Autodesk Fusion 360 part; units mm, degrees
(part 2 of 2)
sketch "Skizze22" plane through (0, 0, 0) normal (0, 1, 0) x (1, 0, 0)
  circle A0 centre (300.5747, -360.375) radius 1.05
  circle A1 centre (290.8247, -423.625) radius 1.05
  circle A2 centre (342.5747, -360.375) radius 1.05
  circle A3 centre (300.5747, -410.375) radius 1.05
  circle A4 centre (352.3247, -423.625) radius 1.05
  circle A5 centre (290.8247, -347.125) radius 1.05
  circle A6 centre (342.5747, -410.375) radius 1.05
  circle A7 centre (352.3247, -347.125) radius 1.05
  line L0 (372.375, -423.1301) -> (372.375, -432.6968)
  line L1 (372.375, -443.625) -> (354.375, -443.625)
  line L2 (270.8247, -443.625) -> (270.8247, -437.3156)
  line L3 (270.8247, -437.3156) -> (274.8247, -439.625)
  line L4 (274.8247, -439.625) -> (278.8247, -437.3156)
  line L5 (278.8247, -437.3156) -> (278.8247, -432.6968)
  line L6 (278.8247, -432.6968) -> (274.8247, -430.3874)
  line L7 (274.8247, -430.3874) -> (270.8247, -432.6968)
  line L8 (270.8247, -432.6968) -> (270.8247, -423.1299)
  line L9 (270.8247, -333.4429) -> (270.8247, -327.125)
  line L10 (270.8247, -327.125) -> (288.875, -327.125)
  line L11 (372.375, -327.125) -> (372.375, -333.4372)
  line L12 (372.375, -338.0617) -> (372.375, -347.6245)
  line L13 (372.375, -347.6245) -> (365.5189, -347.6245)
  line L14 (365.5189, -347.6245) -> (352.7821, -385.3833)
  line L15 (352.7821, -385.3833) -> (365.5137, -423.1301)
  line L16 (365.5137, -423.1301) -> (372.375, -423.1301)
  circle A8 centre (352.3247, -347.125) radius 1.05
  circle A9 centre (342.5747, -410.375) radius 1.05
  circle A10 centre (290.8247, -347.125) radius 1.05
  circle A11 centre (352.3247, -423.625) radius 1.05
  circle A12 centre (300.5747, -410.375) radius 1.05
  circle A13 centre (342.5747, -360.375) radius 1.05
  circle A14 centre (290.8247, -423.625) radius 1.05
  circle A15 centre (300.5747, -360.375) radius 1.05
  line L17 (354.375, -443.625) -> (372.375, -443.625)
  line L18 (270.8247, -437.3156) -> (270.8247, -443.625)
  line L19 (270.8247, -437.3156) -> (274.8247, -439.625)
  line L20 (274.8247, -439.625) -> (278.8247, -437.3156)
  line L21 (278.8247, -437.3156) -> (278.8247, -432.6968)
  line L22 (278.8247, -432.6968) -> (274.8247, -430.3874)
  line L23 (274.8247, -430.3874) -> (270.8247, -432.6968)
  line L24 (270.8247, -423.1299) -> (270.8247, -432.6968)
  line L25 (270.8247, -327.125) -> (270.8247, -333.4429)
  line L26 (288.875, -327.125) -> (270.8247, -327.125)
  line L27 (372.375, -333.4372) -> (372.375, -327.125)
  line L28 (372.375, -347.6245) -> (372.375, -338.0617)
  line L29 (365.5189, -347.6245) -> (372.375, -347.6245)
  line L30 (352.7821, -385.3833) -> (365.5189, -347.6245)
  line L31 (365.5137, -423.1301) -> (352.7821, -385.3833)
  line L32 (372.375, -423.1301) -> (365.5137, -423.1301)
  line L33 (372.375, -432.6968) -> (372.375, -423.1301)
  line L34 (372.375, -333.4372) -> (376.3602, -331.125)
  line L35 (376.3602, -331.125) -> (380.3651, -333.4259)
  line L36 (380.3651, -333.4259) -> (380.375, -338.0447)
  line L37 (380.375, -338.0447) -> (376.3799, -340.3626)
  line L38 (376.3799, -340.3626) -> (372.375, -338.0617)
  arc A16 (176.5, -116.5) -> (180.5, -112.5) centre (180.5, -116.5) ccw
  line L39 (176.5, -116.5) -> (71.5, -116.5)
  arc A17 (67.5, -112.5) -> (71.5, -116.5) centre (67.5, -116.5) ccw
  line L40 (67.5, -112.5) -> (67.5, -95)
  arc A18 (67.5, -87) -> (67.5, -95) centre (67.5, -91) ccw
  line L41 (67.5, -87) -> (67.5, -69)
  arc A19 (71.5, -65) -> (67.5, -69) centre (67.5, -65) ccw
  line L42 (71.5, -65) -> (176.5, -65)
  arc A20 (180.5, -69) -> (176.5, -65) centre (180.5, -65) ccw
  line L43 (180.5, -69) -> (180.5, -87)
  arc A21 (180.5, -95) -> (180.5, -87) centre (180.5, -91) ccw
  line L44 (180.5, -95) -> (180.5, -112.5)
  line L45 (137.5, 7.5) -> (104.5, 7.5)
  line L46 (104.5, 7.5) -> (104.5, 23.5)
  line L47 (104.5, 23.5) -> (102, 23.5)
  line L48 (102, 23.5) -> (102, 34.5)
  line L49 (102, 34.5) -> (140, 34.5)
  line L50 (140, 34.5) -> (140, 23.5)
  line L51 (140, 23.5) -> (137.5, 23.5)
  line L52 (137.5, 23.5) -> (137.5, 7.5)
  line L53 (455, -207) -> (552.928, -207)
  line L54 (552.928, -207) -> (552.928, -27)
  line L55 (552.928, -27) -> (455, -27)
  line L56 (455, -27) -> (455, -207)
  line L57 (583, -14) -> (583, -27)
  line L58 (583, -27) -> (572.928, -27)
  line L59 (572.928, -27) -> (572.928, -207)
  line L60 (572.928, -207) -> (583, -207)
  line L61 (583, -207) -> (583, -225)
  line L62 (583, -225) -> (315, -225)
  line L63 (315, -225) -> (315, -14)
  line L64 (315, -14) -> (583, -14)
  line L65 (59, -3.5) -> (35, -3.5)
  line L66 (35, -3.5) -> (35, 34.5)
  line L67 (35, 34.5) -> (59, 34.5)
  line L68 (59, 34.5) -> (59, -3.5)
  line L69 (82, 4.5) -> (82, 34.5)
  line L70 (82, 34.5) -> (100, 34.5)
  line L71 (100, 34.5) -> (100, 4.5)
  line L72 (100, 4.5) -> (82, 4.5)
  circle A22 centre (386.2786, 261.3333) radius 3
  circle A23 centre (386.2786, 178.3693) radius 2
  line L73 (382.7786, 285.8333) -> (389.7786, 285.8333)
  line L74 (389.7786, 285.8333) -> (389.7786, 271.3333)
  line L75 (389.7786, 271.3333) -> (382.7786, 271.3333)
  line L76 (382.7786, 271.3333) -> (382.7786, 285.8333)
  line L77 (-65.5, -219) -> (-65.5, -239)
  line L78 (-65.5, -239) -> (-66.5, -239)
  line L79 (-66.5, -239) -> (-66.5, -219)
  line L80 (-66.5, -219) -> (-65.5, -219)
  circle A24 centre (115, 170.025) radius 2
  circle A25 centre (220, 275.025) radius 2
  circle A26 centre (115, 275.025) radius 2
  circle A27 centre (167.5, 222.525) radius 57.5
  circle A28 centre (220, 170.025) radius 2
  line L81 (92.5, 328.025) -> (242.5, 328.025)
  line L82 (242.5, 328.025) -> (242.5, 117.025)
  line L83 (242.5, 117.025) -> (92.5, 117.025)
  line L84 (92.5, 117.025) -> (92.5, 328.025)
  circle A29 centre (22, 160.025) radius 2
  circle A30 centre (-102, 160.025) radius 2
  circle A31 centre (-102, 284.025) radius 2
  circle A32 centre (22, 284.025) radius 2
  circle A33 centre (-40, 222.025) radius 67.5
  line L85 (-115, 327.525) -> (35, 327.525)
  line L86 (35, 327.525) -> (35, 116.525)
  line L87 (35, 116.525) -> (-115, 116.525)
  line L88 (-115, 116.525) -> (-115, 327.525)
  line L89 (190.5, -319) -> (190.5, -339)
  line L90 (190.5, -339) -> (189.5, -339)
  line L91 (189.5, -339) -> (189.5, -319)
  line L92 (189.5, -319) -> (190.5, -319)
  line L93 (198, -317) -> (182, -317)
  line L94 (182, -317) -> (182, -339.5)
  line L95 (182, -339.5) -> (-58, -339.5)
  line L96 (-58, -339.5) -> (-58, -219.5)
  line L97 (-58, -219.5) -> (182, -219.5)
  line L98 (182, -219.5) -> (182, -242)
  line L99 (182, -242) -> (198, -242)
  arc A34 (203, -247) -> (198, -242) centre (198, -247) ccw
  line L100 (203, -247) -> (203, -312)
  arc A35 (198, -317) -> (203, -312) centre (198, -312) ccw
  line L101 (382.7786, 235.3333) -> (389.7786, 235.3333)
  line L102 (389.7786, 235.3333) -> (389.7786, 220.8333)
  line L103 (389.7786, 220.8333) -> (382.7786, 220.8333)
  line L104 (382.7786, 220.8333) -> (382.7786, 235.3333)
  circle A36 centre (386.283, 172.3693) radius 3.5
  circle A37 centre (386.2786, 245.3333) radius 3
  circle A38 centre (386.2786, 162.3693) radius 4.5
  line L105 (78.5, 4.5) -> (60.5, 4.5)
  line L106 (60.5, 4.5) -> (60.5, 34.5)
  line L107 (60.5, 34.5) -> (78.5, 34.5)
  line L108 (78.5, 34.5) -> (78.5, 4.5)
  line L109 (28.5, 32) -> (28.5, -74)
  line L110 (28.5, -74) -> (35.5, -74)
  line L111 (35.5, -74) -> (35.5, -77)
  line L112 (35.5, -77) -> (-15.5, -77)
  line L113 (-15.5, -77) -> (-15.5, -74)
  line L114 (-15.5, -74) -> (-8.5, -74)
  line L115 (-8.5, -74) -> (-8.5, 32)
  line L116 (-8.5, 32) -> (28.5, 32)
  circle A39 centre (300.5747, -410.375) radius 1.05
  circle A40 centre (342.5747, -360.375) radius 1.05
  circle A41 centre (352.3247, -347.125) radius 1.05
  circle A42 centre (342.5747, -410.375) radius 1.05
  circle A43 centre (300.5747, -360.375) radius 1.05
  circle A44 centre (290.8247, -423.625) radius 1.05
  circle A45 centre (352.3247, -423.625) radius 1.05
  circle A46 centre (290.8247, -347.125) radius 1.05
  line L117 (270.8247, -443.625) -> (270.8247, -437.3156)
  line L118 (270.8247, -437.3156) -> (274.8247, -439.625)
  line L119 (274.8247, -439.625) -> (278.8247, -437.3156)
  line L120 (278.8247, -437.3156) -> (278.8247, -432.6968)
  line L121 (278.8247, -432.6968) -> (274.8247, -430.3874)
  line L122 (274.8247, -430.3874) -> (270.8247, -432.6968)
  line L123 (270.8247, -432.6968) -> (270.8247, -423.1299)
  line L124 (270.8247, -333.4429) -> (270.8247, -327.125)
  line L125 (270.8247, -327.125) -> (288.875, -327.125)
  line L126 (372.375, -327.125) -> (372.375, -333.4372)
  line L127 (372.375, -333.4372) -> (376.3602, -331.125)
  line L128 (376.3602, -331.125) -> (380.3651, -333.4259)
  line L129 (380.3651, -333.4259) -> (380.375, -338.0447)
  line L130 (380.375, -338.0447) -> (376.3799, -340.3626)
  line L131 (376.3799, -340.3626) -> (372.375, -338.0617)
  line L132 (372.375, -338.0617) -> (372.375, -347.6245)
  line L133 (372.375, -347.6245) -> (365.5189, -347.6245)
  line L134 (365.5189, -347.6245) -> (352.7821, -385.3833)
  line L135 (352.7821, -385.3833) -> (365.5137, -423.1301)
  line L136 (365.5137, -423.1301) -> (372.375, -423.1301)
  line L137 (372.375, -423.1301) -> (372.375, -432.6968)
  line L138 (372.375, -443.625) -> (354.375, -443.625)
  line L139 (-66.5, -319) -> (-65.5, -319)
  line L140 (-65.5, -319) -> (-65.5, -339)
  line L141 (-65.5, -339) -> (-66.5, -339)
  line L142 (-66.5, -339) -> (-66.5, -319)
  line L143 (189.5, -239) -> (189.5, -219)
  line L144 (189.5, -219) -> (190.5, -219)
  line L145 (190.5, -219) -> (190.5, -239)
  line L146 (190.5, -239) -> (189.5, -239)
  arc A47 (176.5, -116.5) -> (180.5, -112.5) centre (180.5, -116.5) ccw
  line L147 (176.5, -116.5) -> (71.5, -116.5)
  arc A48 (67.5, -112.5) -> (71.5, -116.5) centre (67.5, -116.5) ccw
  line L148 (67.5, -112.5) -> (67.5, -95)
  arc A49 (67.5, -87) -> (67.5, -95) centre (67.5, -91) ccw
  line L149 (67.5, -87) -> (67.5, -69)
  arc A50 (71.5, -65) -> (67.5, -69) centre (67.5, -65) ccw
  line L150 (71.5, -65) -> (176.5, -65)
  arc A51 (180.5, -69) -> (176.5, -65) centre (180.5, -65) ccw
  line L151 (180.5, -69) -> (180.5, -87)
  arc A52 (180.5, -95) -> (180.5, -87) centre (180.5, -91) ccw
  line L152 (180.5, -95) -> (180.5, -112.5)
  line L153 (137.5, 7.5) -> (104.5, 7.5)
  line L154 (104.5, 7.5) -> (104.5, 23.5)
  line L155 (104.5, 23.5) -> (102, 23.5)
  line L156 (102, 23.5) -> (102, 34.5)
  line L157 (102, 34.5) -> (140, 34.5)
  line L158 (140, 34.5) -> (140, 23.5)
  line L159 (140, 23.5) -> (137.5, 23.5)
  line L160 (137.5, 23.5) -> (137.5, 7.5)
  line L161 (455, -207) -> (552.928, -207)
  line L162 (552.928, -207) -> (552.928, -27)
  line L163 (552.928, -27) -> (455, -27)
  line L164 (455, -27) -> (455, -207)
  line L165 (583, -14) -> (583, -27)
  line L166 (583, -27) -> (572.928, -27)
  line L167 (572.928, -27) -> (572.928, -207)
  line L168 (572.928, -207) -> (583, -207)
  line L169 (583, -207) -> (583, -225)
  line L170 (583, -225) -> (315, -225)
  line L171 (315, -225) -> (315, -14)
  line L172 (315, -14) -> (583, -14)
  line L173 (59, -3.5) -> (35, -3.5)
  line L174 (35, -3.5) -> (35, 34.5)
  line L175 (35, 34.5) -> (59, 34.5)
  line L176 (59, 34.5) -> (59, -3.5)
  line L177 (82, 4.5) -> (82, 34.5)
  line L178 (82, 34.5) -> (100, 34.5)
  line L179 (100, 34.5) -> (100, 4.5)
  line L180 (100, 4.5) -> (82, 4.5)
  circle A53 centre (386.2786, 261.3333) radius 3
  circle A54 centre (386.2786, 178.3693) radius 2
  line L181 (382.7786, 285.8333) -> (389.7786, 285.8333)
  line L182 (389.7786, 285.8333) -> (389.7786, 271.3333)
  line L183 (389.7786, 271.3333) -> (382.7786, 271.3333)
  line L184 (382.7786, 271.3333) -> (382.7786, 285.8333)
  line L185 (-65.5, -219) -> (-65.5, -239)
  line L186 (-65.5, -239) -> (-66.5, -239)
  line L187 (-66.5, -239) -> (-66.5, -219)
  line L188 (-66.5, -219) -> (-65.5, -219)
  circle A55 centre (115, 170.025) radius 2
  circle A56 centre (220, 275.025) radius 2
  circle A57 centre (115, 275.025) radius 2
  circle A58 centre (167.5, 222.525) radius 57.5
  circle A59 centre (220, 170.025) radius 2
  line L189 (92.5, 328.025) -> (242.5, 328.025)
  line L190 (242.5, 328.025) -> (242.5, 117.025)
  line L191 (242.5, 117.025) -> (92.5, 117.025)
  line L192 (92.5, 117.025) -> (92.5, 328.025)
  circle A60 centre (22, 160.025) radius 2
  circle A61 centre (-102, 160.025) radius 2
  circle A62 centre (-102, 284.025) radius 2
  circle A63 centre (22, 284.025) radius 2
  circle A64 centre (-40, 222.025) radius 67.5
  line L193 (-115, 327.525) -> (35, 327.525)
  line L194 (35, 327.525) -> (35, 116.525)
  line L195 (35, 116.525) -> (-115, 116.525)
  line L196 (-115, 116.525) -> (-115, 327.525)
  line L197 (190.5, -319) -> (190.5, -339)
  line L198 (190.5, -339) -> (189.5, -339)
  line L199 (189.5, -339) -> (189.5, -319)
  line L200 (189.5, -319) -> (190.5, -319)
  line L201 (198, -317) -> (182, -317)
  line L202 (182, -317) -> (182, -339.5)
  line L203 (182, -339.5) -> (-58, -339.5)
  line L204 (-58, -339.5) -> (-58, -219.5)
  line L205 (-58, -219.5) -> (182, -219.5)
  line L206 (182, -219.5) -> (182, -242)
  line L207 (182, -242) -> (198, -242)
  arc A65 (203, -247) -> (198, -242) centre (198, -247) ccw
  line L208 (203, -247) -> (203, -312)
  arc A66 (198, -317) -> (203, -312) centre (198, -312) ccw
  line L209 (382.7786, 235.3333) -> (389.7786, 235.3333)
  line L210 (389.7786, 235.3333) -> (389.7786, 220.8333)
  line L211 (389.7786, 220.8333) -> (382.7786, 220.8333)
  line L212 (382.7786, 220.8333) -> (382.7786, 235.3333)
  circle A67 centre (386.283, 172.3693) radius 3.5
  circle A68 centre (386.2786, 245.3333) radius 3
  circle A69 centre (386.2786, 162.3693) radius 4.5
  line L213 (78.5, 4.5) -> (60.5, 4.5)
  line L214 (60.5, 4.5) -> (60.5, 34.5)
  line L215 (60.5, 34.5) -> (78.5, 34.5)
  line L216 (78.5, 34.5) -> (78.5, 4.5)
  line L217 (28.5, 32) -> (28.5, -74)
  line L218 (28.5, -74) -> (35.5, -74)
  line L219 (35.5, -74) -> (35.5, -77)
  line L220 (35.5, -77) -> (-15.5, -77)
  line L221 (-15.5, -77) -> (-15.5, -74)
  line L222 (-15.5, -74) -> (-8.5, -74)
  line L223 (-8.5, -74) -> (-8.5, 32)
  line L224 (-8.5, 32) -> (28.5, 32)
  circle A70 centre (300.5747, -410.375) radius 1.05
  circle A71 centre (342.5747, -360.375) radius 1.05
  circle A72 centre (352.3247, -347.125) radius 1.05
  circle A73 centre (342.5747, -410.375) radius 1.05
  circle A74 centre (300.5747, -360.375) radius 1.05
  circle A75 centre (290.8247, -423.625) radius 1.05
  circle A76 centre (352.3247, -423.625) radius 1.05
  circle A77 centre (290.8247, -347.125) radius 1.05
  line L225 (270.8247, -443.625) -> (270.8247, -437.3156)
  line L226 (270.8247, -437.3156) -> (274.8247, -439.625)
  line L227 (274.8247, -439.625) -> (278.8247, -437.3156)
  line L228 (278.8247, -437.3156) -> (278.8247, -432.6968)
  line L229 (278.8247, -432.6968) -> (274.8247, -430.3874)
  line L230 (274.8247, -430.3874) -> (270.8247, -432.6968)
  line L231 (270.8247, -432.6968) -> (270.8247, -423.1299)
  line L232 (270.8247, -333.4429) -> (270.8247, -327.125)
  line L233 (270.8247, -327.125) -> (288.875, -327.125)
  line L234 (372.375, -327.125) -> (372.375, -333.4372)
  line L235 (372.375, -333.4372) -> (376.3602, -331.125)
  line L236 (376.3602, -331.125) -> (380.3651, -333.4259)
  line L237 (380.3651, -333.4259) -> (380.375, -338.0447)
  line L238 (380.375, -338.0447) -> (376.3799, -340.3626)
  line L239 (376.3799, -340.3626) -> (372.375, -338.0617)
  line L240 (372.375, -338.0617) -> (372.375, -347.6245)
  line L241 (372.375, -347.6245) -> (365.5189, -347.6245)
  line L242 (365.5189, -347.6245) -> (352.7821, -385.3833)
  line L243 (352.7821, -385.3833) -> (365.5137, -423.1301)
  line L244 (365.5137, -423.1301) -> (372.375, -423.1301)
  line L245 (372.375, -423.1301) -> (372.375, -432.6968)
  line L246 (372.375, -443.625) -> (354.375, -443.625)
  line L247 (-66.5, -319) -> (-65.5, -319)
  line L248 (-65.5, -319) -> (-65.5, -339)
  line L249 (-65.5, -339) -> (-66.5, -339)
  line L250 (-66.5, -339) -> (-66.5, -319)
  line L251 (189.5, -239) -> (189.5, -219)
  line L252 (189.5, -219) -> (190.5, -219)
  line L253 (190.5, -219) -> (190.5, -239)
  line L254 (190.5, -239) -> (189.5, -239)
  line L255 (376.3602, -331.125) -> (372.375, -333.4372)
  line L256 (380.3651, -333.4259) -> (376.3602, -331.125)
  line L257 (380.375, -338.0447) -> (380.3651, -333.4259)
  line L258 (376.3799, -340.3626) -> (380.375, -338.0447)
  line L259 (372.375, -338.0617) -> (376.3799, -340.3626)
  line L260 (274.8394, -340.3626) -> (278.8345, -338.0447)
  line L261 (278.8345, -338.0447) -> (278.8247, -333.4259)
  line L262 (278.8247, -333.4259) -> (274.8198, -331.125)
  line L263 (274.8198, -331.125) -> (270.8247, -333.4429)
  line L264 (270.8247, -333.4429) -> (270.8345, -338.0617)
  line L265 (270.8345, -338.0617) -> (274.8394, -340.3626)
  line L266 (372.375, -432.6968) -> (376.375, -430.3874)
  line L267 (376.375, -430.3874) -> (380.375, -432.6968)
  line L268 (380.375, -432.6968) -> (380.375, -437.3156)
  line L269 (380.375, -437.3156) -> (376.375, -439.625)
  line L270 (376.375, -439.625) -> (372.375, -437.3156)
  line L271 (372.375, -437.3156) -> (372.375, -443.625)
  line L272 (274.8394, -340.3626) -> (278.8345, -338.0447)
  line L273 (278.8345, -338.0447) -> (278.8247, -333.4259)
  line L274 (278.8247, -333.4259) -> (274.8198, -331.125)
  line L275 (274.8198, -331.125) -> (270.8247, -333.4429)
  line L276 (270.8247, -333.4429) -> (270.8345, -338.0617)
  line L277 (270.8345, -338.0617) -> (274.8394, -340.3626)
  line L278 (372.375, -432.6968) -> (376.375, -430.3874)
  line L279 (376.375, -430.3874) -> (380.375, -432.6968)
  line L280 (380.375, -432.6968) -> (380.375, -437.3156)
  line L281 (380.375, -437.3156) -> (376.375, -439.625)
  line L282 (376.375, -439.625) -> (372.375, -437.3156)
  line L283 (372.375, -437.3156) -> (372.375, -443.625)
  line L284 (274.8394, -340.3626) -> (278.8345, -338.0447)
  line L285 (278.8345, -338.0447) -> (278.8247, -333.4259)
  line L286 (278.8247, -333.4259) -> (274.8198, -331.125)
  line L287 (274.8198, -331.125) -> (270.8247, -333.4429)
  line L288 (270.8247, -333.4429) -> (270.8345, -338.0617)
  line L289 (270.8345, -338.0617) -> (274.8394, -340.3626)
  line L290 (372.375, -432.6968) -> (376.375, -430.3874)
  line L291 (376.375, -430.3874) -> (380.375, -432.6968)
  line L292 (380.375, -432.6968) -> (380.375, -437.3156)
  line L293 (380.375, -437.3156) -> (376.375, -439.625)
  line L294 (376.375, -439.625) -> (372.375, -437.3156)
  line L295 (372.375, -437.3156) -> (372.375, -443.625)
  line L296 (278.8345, -338.0447) -> (278.8247, -333.4259)
  line L297 (278.8247, -333.4259) -> (274.8198, -331.125)
  line L298 (274.8198, -331.125) -> (270.8247, -333.4429)
  line L299 (270.8247, -333.4429) -> (270.8345, -338.0617)
  line L300 (270.8345, -338.0617) -> (274.8394, -340.3626)
  line L301 (274.8394, -340.3626) -> (278.8345, -338.0447)
  line L302 (376.375, -430.3874) -> (372.375, -432.6968)
  line L303 (380.375, -432.6968) -> (376.375, -430.3874)
  line L304 (380.375, -437.3156) -> (380.375, -432.6968)
  line L305 (376.375, -439.625) -> (380.375, -437.3156)
  line L306 (372.375, -437.3156) -> (376.375, -439.625)
  line L307 (372.375, -443.625) -> (372.375, -437.3156)
  line L308 (270.8247, -423.1299) -> (277.6357, -423.1301)
  line L309 (277.6357, -423.1301) -> (290.3673, -385.3833)
  line L310 (290.3673, -385.3833) -> (277.6305, -347.6245)
  line L311 (277.6305, -347.6245) -> (270.8247, -347.6245)
  line L312 (270.8247, -347.6245) -> (270.8247, -333.4429)
  line L313 (288.875, -327.125) -> (288.875, -336.084)
  line L314 (288.875, -336.084) -> (321.625, -343.6621)
  line L315 (321.625, -343.6621) -> (354.375, -336.084)
  line L316 (354.375, -336.084) -> (354.375, -327.125)
  line L317 (354.375, -327.125) -> (372.375, -327.125)
  line L318 (354.375, -443.625) -> (354.375, -434.666)
  line L319 (354.375, -434.666) -> (321.625, -427.088)
  line L320 (321.625, -427.088) -> (288.875, -434.666)
  line L321 (288.875, -434.666) -> (288.875, -443.625)
  line L322 (288.875, -443.625) -> (270.8247, -443.625)
  line L323 (270.8247, -423.1299) -> (277.6357, -423.1301)
  line L324 (277.6357, -423.1301) -> (290.3673, -385.3833)
  line L325 (290.3673, -385.3833) -> (277.6305, -347.6245)
  line L326 (277.6305, -347.6245) -> (270.8247, -347.6245)
  line L327 (270.8247, -347.6245) -> (270.8247, -333.4429)
  line L328 (288.875, -327.125) -> (288.875, -336.084)
  line L329 (288.875, -336.084) -> (321.625, -343.6621)
  line L330 (321.625, -343.6621) -> (354.375, -336.084)
  line L331 (354.375, -336.084) -> (354.375, -327.125)
  line L332 (354.375, -327.125) -> (372.375, -327.125)
  line L333 (354.375, -443.625) -> (354.375, -434.666)
  line L334 (354.375, -434.666) -> (321.625, -427.088)
  line L335 (321.625, -427.088) -> (288.875, -434.666)
  line L336 (288.875, -434.666) -> (288.875, -443.625)
  line L337 (288.875, -443.625) -> (270.8247, -443.625)
  line L338 (270.8247, -423.1299) -> (277.6357, -423.1301)
  line L339 (277.6357, -423.1301) -> (290.3673, -385.3833)
  line L340 (290.3673, -385.3833) -> (277.6305, -347.6245)
  line L341 (277.6305, -347.6245) -> (270.8247, -347.6245)
  line L342 (270.8247, -347.6245) -> (270.8247, -333.4429)
  line L343 (288.875, -327.125) -> (288.875, -336.084)
  line L344 (288.875, -336.084) -> (321.625, -343.6621)
  line L345 (321.625, -343.6621) -> (354.375, -336.084)
  line L346 (354.375, -336.084) -> (354.375, -327.125)
  line L347 (354.375, -327.125) -> (372.375, -327.125)
  line L348 (354.375, -443.625) -> (354.375, -434.666)
  line L349 (354.375, -434.666) -> (321.625, -427.088)
  line L350 (321.625, -427.088) -> (288.875, -434.666)
  line L351 (288.875, -434.666) -> (288.875, -443.625)
  line L352 (288.875, -443.625) -> (270.8247, -443.625)
  line L353 (270.8247, -423.1299) -> (277.6357, -423.1301)
  line L354 (277.6357, -423.1301) -> (290.3673, -385.3833)
  line L355 (290.3673, -385.3833) -> (277.6305, -347.6245)
  line L356 (277.6305, -347.6245) -> (270.8247, -347.6245)
  line L357 (270.8247, -333.4429) -> (270.8247, -347.6245)
  line L358 (288.875, -336.084) -> (288.875, -327.125)
  line L359 (321.625, -343.6621) -> (288.875, -336.084)
  line L360 (354.375, -336.084) -> (321.625, -343.6621)
  line L361 (354.375, -327.125) -> (354.375, -336.084)
  line L362 (372.375, -327.125) -> (354.375, -327.125)
  line L363 (354.375, -443.625) -> (354.375, -434.666)
  line L364 (354.375, -434.666) -> (321.625, -427.088)
  line L365 (321.625, -427.088) -> (288.875, -434.666)
  line L366 (288.875, -434.666) -> (288.875, -443.625)
  line L367 (270.8247, -443.625) -> (288.875, -443.625)
equation "d68 = 400 mm - 36 mm"
equation "d69 = width"
equation "d72 = ( width - 120 mm ) / 2"
equation "d76 = ( ( 120 - 75 ) / 2 ) * 1 mm"
equation "d79 = width"
equation "d81 = width"
equation "d84 = width / 2"
equation "d85 = width / 2"
equation "d86 = ( 150 / 2 ) * 1 mm"
equation "d87 = ( 150 / 2 ) * 1 mm"
equation "d98 = ( 124 / 2 ) * 1 mm"
equation "d99 = ( 124 / 2 ) * 1 mm"
equation "d105 = width"
equation "d130 = ( ( 42 - 15 ) / 2 ) * 1 mm"
equation "d131 = ( ( 42 - 30 ) / 2 ) * 1 mm"
equation "d134 = ( width - 100 mm ) / 3"
equation "d138 = ( width - 100 mm ) / 3"
equation "d160 = width"
equation "nx = 5"
equation "ny = 5"
equation "d200 = standoff_diam"
equation "d201 = standoff_diam"
equation "d202 = standoff_diam"
equation "d203 = standoff_diam"
equation "d207 = standoff_diam"
equation "d208 = standoff_diam"
equation "d209 = standoff_diam"
equation "d210 = ( ( 61.5 - 42 ) / 2 ) * 1 mm"
equation "d211 = ( ( 76.5 - 50 ) / 2 ) * 1 mm"
equation "d220 = ( 42 / 2 ) * 1 mm"
equation "d223 = ( 50 / 2 ) * 1 mm"
named bodies: "back"
